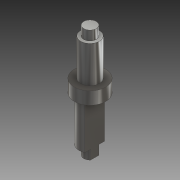
# Autodesk Inventor part: thumb_03 IP shaft
Saved by Autodesk Inventor 2017 SP1 (Build 210196100, 196)
## iProperties
Created: 2017-06-05
Part Number: thumb_03 IP shaft
Material: Generic
Document SubType Name: Modeling
Designer: Tomasz
Density: 1 g/cm^3
Appearance: Steel - Polished
Author: Tomasz
Autodesk Inventor part; units mm, degrees
ref_plane "YZ Plane" through (0, 0, 0) normal (1, 0, 0) x (0, 1, 0)
ref_plane "XZ Plane" through (0, 0, 0) normal (0, 1, 0) x (-1, 0, 0)
ref_plane "XY Plane" through (0, 0, 0) normal (0, 0, 1) x (1, 0, 0)
sketch "Sketch1" plane through (0, 0, 0) normal (0, 1, 0) x (-1, 0, 0)
  line L0 (0, 0) -> (1, 0)
  line L1 (1, 0) -> (1, -1.5)
  line L2 (1, -1.5) -> (1.5, -1.5)
  line L3 (1.5, -7.35) -> (2.5, -7.35)
  line L4 (2.5, -7.35) -> (2.5, -9.35)
  line L5 (2.5, -9.35) -> (1.75, -9.35)
  line L6 (1.75, -9.35) -> (1.75, -16.5)
  line L7 (1, -18) -> (0, -18)
  line L8 (0, 0) -> (0, -18)
  line L9 (1.4788, -16.5) -> (1, -16.5)
  line L10 (1, -16.5) -> (1, -18)
  line L11 (1.4788, -16.5) -> (1.75, -16.5)
  line L12 (1.5, -1.5) -> (1.5, -7.35)
  line L13 (1.5, -7.35) -> (1.5, -1.5)
  dimension "d1" = 1.5
  dimension "d19" = 15
  dimension "d21" = 1.5
  dimension "d30" = 2
  dimension "d31" = 2
  dimension "d33" = 3.5
  dimension "d34" = 5
  dimension "d35" = 3
  dimension "d47" = 5.85
  dimension "d48" = 2
  constraints: 28 end point, 5 perpendicular, 3 horizontal, 3 point on line, 2 vertical, 1 coincident, 2 other
  measures "d1" distance between parallel lines of L2 L0
  measures "d19" distance between parallel lines of L9 L2
  measures "d21" distance between parallel lines of L9 L7
  measures "d30" diameter of L1 L8
  measures "d31" diameter of L10 L8
  measures "d33" diameter of L6 L8
  measures "d34" diameter of L4 L8
  measures "d35" diameter of L12 L8
  measures "d47" distance between parallel lines of L3 L2
  measures "d48" distance between parallel lines of L5 L3
revolve "Revolution1" add sketch "Sketch1" angle 360 about axis through (0, 0, 0) along (0, 0, -1)
sketch "Sketch4" plane through (0, 0, -18) normal (0, 0, -1) x (-1, 0, 0)
  circle A0 centre (0, 0) radius 1.75 projected
  line L0 (-0.75, -1.5811) -> (-0.75, 1.5811)
  dimension "d43" = 0.75
  constraints: 2 end point, 2 point on circle, 1 vertical
  measures "d43" distance from line of A0.centre L0
extrude "Extrusion1" cut sketch "Sketch4" against normal up to surface (8.65 mm away) contours L0 A0 picked at (-1.0833, 0)
body "Solid1"
